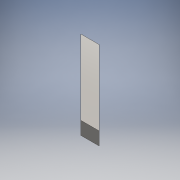
# Autodesk Inventor part: Truss for cantilever
Saved by Autodesk Inventor 2016 (Build 200138000, 138)
## iProperties
Created: 2019-03-24
Part Number: Truss for cantilever
Material: Stainless Steel
Document SubType Name: Modeling
Designer: benja
Density: 8 g/cm^3
Appearance: Semi-Polished
Author: benja
Autodesk Inventor part; units mm, degrees
ref_plane "YZ Plane" through (0, 0, 0) normal (1, 0, 0) x (0, 1, 0)
ref_plane "XZ Plane" through (0, 0, 0) normal (0, 1, 0) x (-1, 0, 0)
ref_plane "XY Plane" through (0, 0, 0) normal (0, 0, 1) x (1, 0, 0)
sketch "Sketch1" plane through (0, 0, 0) normal (0, 0, 1) x (1, 0, 0)
  line L0 (0, 0) -> (0, 800)
  line L1 (0, 800) -> (800, 0)
  line L2 (197.9899, 800) -> (997.9899, 0)
  line L3 (0, 800) -> (197.9899, 800)
  line L4 (800, 0) -> (997.9899, 0)
  dimension "d0" = 800
  dimension "d1" = 45
  dimension "d3" = 140
  constraints: 10 end point, 2 parallel, 1 horizontal, 1 vertical
  measures "d0" distance of L0.start L0.end
  measures "d1" angle of L0 L1
  measures "d3" distance between parallel lines of L2 L1
extrude "Extrusion1" add sketch "Sketch1" along normal blind 140
body "Solid1"
